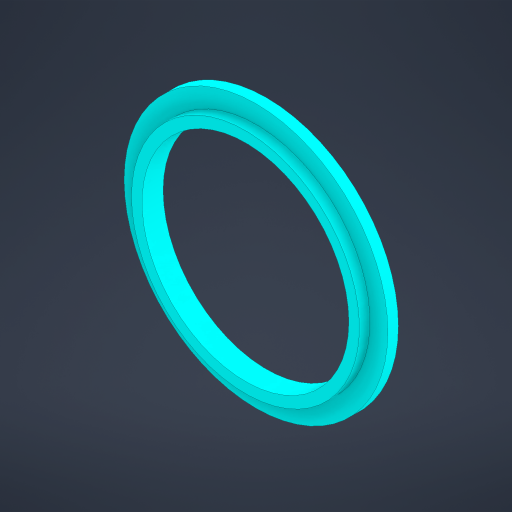
# Autodesk Inventor part: One Inch Lense Holder Cover (V5)
Saved by Autodesk Inventor 2023.4 (Build 274418000, 418)
## iProperties
Created: 2024-04-25
Part Number: One Inch Lense Holder Cover (V5)
Material: Generic
Document SubType Name: Modeling
Designer: xSibe
Density: 1 g/cm^3
Appearance: Plastic Cyan
Author: xSibe
Autodesk Inventor part; units mm, degrees
ref_plane "YZ Plane" through (0, 0, 0) normal (1, 0, 0) x (0, 1, 0)
ref_plane "XZ Plane" through (0, 0, 0) normal (0, 1, 0) x (-1, 0, 0)
sketch "Sketch1" plane through (0, 0, 0) normal (0, 0, 1) x (1, 0, 0)
  circle A0 centre (1.767767, 26.667767) radius 13.575
  circle A1 centre (1.767767, 26.667767) radius 13.5375
  circle A2 centre (1.767767, 26.667767) radius 12.2875
  point P0 (0, 0)
  dimension "d0" = 0.0375
  dimension "d1" = 1.25
  constraints: 2 centre point
  measures "d0" radial gap between concentric circles of A0 A1
  measures "d1" radial gap between concentric circles of A1 A2
ref_plane "Work Plane1" through (-21.967767, 1.0375, -4.375) normal (0, 0, -1) x (0, 1, 0)
sketch "Sketch1 outline for Extrusion1" plane through (0, 0, 0) normal (0, 0, 1) x (1, 0, 0)
  circle A0 centre (1.767767, 26.667767) radius 13.5375
  circle A1 centre (1.767767, 26.667767) radius 12.2875
extrude "Extrusion1" add sketch "Sketch1 outline for Extrusion1" along normal blind 1.25 from surface at -4.375
sketch "Sketch2" plane through (1.767767, 26.667767, -4.375) normal (0, 0, -1) x (-1, 0, 0)
  circle A0 centre (0, 0) radius 13.5375 projected
  circle A1 centre (0, 0) radius 12.2875 projected
  circle A2 centre (0, 0) radius 13.6625
  circle A3 centre (0, 0) radius 15.6625
  point P0 (1.767767, -26.667767)
  dimension "d4" = 0.125
  dimension "d5" = 2
  constraints: 2 centre point
  measures "d4" radial gap between concentric circles of A0 A2
  measures "d5" radial gap between concentric circles of A2 A3
extrude "Extrusion2" add sketch "Sketch2" along normal blind 1.25 contours A0 | A2 | A3
body "Solid1"
